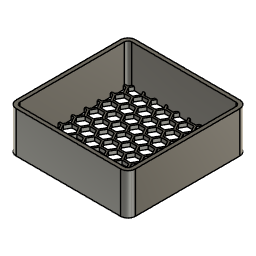
hex napkin holder v1.5 (Autodesk Fusion 360 design; units mm, degrees)
Autodesk Fusion 360 part; units mm, degrees
(part 1 of 14)
sketch "Sketch1" plane through (0, 0, 0) normal (0, 0, 1) x (1, 0, 0)
  line L0 (0, 0) -> (190.5, 0)
  line L1 (190.5, 0) -> (190.5, 190.5)
  line L2 (190.5, 190.5) -> (0, 190.5)
  line L3 (0, 190.5) -> (0, 0)
  line L4 (-6.35, -6.35) -> (196.85, -6.35)
  line L5 (196.85, -6.35) -> (196.85, 196.85)
  line L6 (196.85, 196.85) -> (-6.35, 196.85)
  line L7 (-6.35, 196.85) -> (-6.35, -6.35)
  point P0 (-273.976, 103.1875)
  dimension "d1" = 190.5
  dimension "d2" = 190.5
  dimension "d3" = 6.35
  constraint horizontal L0
  constraint vertical L1
  constraint horizontal L2
  constraint vertical L3
  constraint coincident L0.start L3.end
  measures "d1" distance of L0.start L0.end
  measures "d2" distance of L0.start L2.end
extrude "Extrude1" add sketch "Sketch1" along normal blind 6.35 contours L0 L1 L2 L3
extrude "Extrude2" add sketch "Sketch1" along normal blind 69.85
sketch "Sketch2" plane through (0, 0, 6.35) normal (0, 0, 1) x (-1, 0, 0)
  line L0 (0, -190.5) -> (0, 0)
  line L1 (0, 0) -> (-190.5, 0)
  line L2 (-190.5, 0) -> (-190.5, -190.5)
  line L3 (-190.5, -190.5) -> (0, -190.5)
  line L4 (-190.5, 0) -> (0, -190.5) construction
  line L5 (-190.5, -190.5) -> (0, 0) construction
  line L6 (-100.7493, -104.775) -> (-89.7507, -104.775)
  line L7 (-89.7507, -104.775) -> (-84.2515, -95.25)
  line L8 (-84.2515, -95.25) -> (-89.7507, -85.725)
  line L9 (-89.7507, -85.725) -> (-100.7493, -85.725)
  line L10 (-100.7493, -85.725) -> (-106.2485, -95.25)
  line L11 (-106.2485, -95.25) -> (-100.7493, -104.775)
  line L12 (-95.25, -95.25) -> (-151.2697, -192.279) construction
  line L13 (-95.25, -95.25) -> (-80.5853, -95.25) construction
  line L14 (-95.25, -95.25) -> (-103.4989, -100.0125) construction
  line L15 (-95.25, -95.25) -> (-87.0011, -100.0125) construction
  line L16 (-100.7493, 50.8) -> (-89.7507, 50.8)
  line L17 (-89.7507, 50.8) -> (-84.2515, 60.325)
  line L18 (-84.2515, 60.325) -> (-89.7507, 69.85)
  line L19 (-89.7507, 69.85) -> (-100.7493, 69.85)
  line L20 (-106.2485, 60.325) -> (-100.7493, 50.8)
  line L21 (-100.7493, 69.85) -> (-106.2485, 60.325)
  line L22 (-119.9967, 39.6875) -> (-108.9982, 39.6875)
  line L23 (-108.9982, 39.6875) -> (-103.4989, 49.2125)
  line L24 (-103.4989, 49.2125) -> (-108.9982, 58.7375)
  line L25 (-108.9982, 58.7375) -> (-119.9967, 58.7375)
  line L26 (-125.4959, 49.2125) -> (-119.9967, 39.6875)
  line L27 (-119.9967, 58.7375) -> (-125.4959, 49.2125)
  line L28 (-139.2441, 28.575) -> (-128.2456, 28.575)
  line L29 (-128.2456, 28.575) -> (-122.7463, 38.1)
  line L30 (-122.7463, 38.1) -> (-128.2456, 47.625)
  line L31 (-128.2456, 47.625) -> (-139.2441, 47.625)
  line L32 (-144.7434, 38.1) -> (-139.2441, 28.575)
  line L33 (-139.2441, 47.625) -> (-144.7434, 38.1)
  line L34 (-158.4915, 17.4625) -> (-147.493, 17.4625)
  line L35 (-147.493, 17.4625) -> (-141.9937, 26.9875)
  line L36 (-141.9937, 26.9875) -> (-147.493, 36.5125)
  line L37 (-147.493, 36.5125) -> (-158.4915, 36.5125)
  line L38 (-163.9908, 26.9875) -> (-158.4915, 17.4625)
  line L39 (-158.4915, 36.5125) -> (-163.9908, 26.9875)
  line L40 (-177.7389, 6.35) -> (-166.7404, 6.35)
  line L41 (-166.7404, 6.35) -> (-161.2411, 15.875)
  line L42 (-161.2411, 15.875) -> (-166.7404, 25.4)
  line L43 (-166.7404, 25.4) -> (-177.7389, 25.4)
  line L44 (-183.2382, 15.875) -> (-177.7389, 6.35)
  line L45 (-177.7389, 25.4) -> (-183.2382, 15.875)
  line L46 (-196.9863, -4.7625) -> (-185.9878, -4.7625)
  line L47 (-185.9878, -4.7625) -> (-180.4886, 4.7625)
  line L48 (-180.4886, 4.7625) -> (-185.9878, 14.2875)
  line L49 (-185.9878, 14.2875) -> (-196.9863, 14.2875)
  line L50 (-202.4856, 4.7625) -> (-196.9863, -4.7625)
  line L51 (-196.9863, 14.2875) -> (-202.4856, 4.7625)
  line L52 (-216.2337, -15.875) -> (-205.2352, -15.875)
  line L53 (-205.2352, -15.875) -> (-199.736, -6.35)
  line L54 (-199.736, -6.35) -> (-205.2352, 3.175)
  line L55 (-205.2352, 3.175) -> (-216.2337, 3.175)
  line L56 (-221.733, -6.35) -> (-216.2337, -15.875)
  line L57 (-216.2337, 3.175) -> (-221.733, -6.35)
  line L58 (-235.4812, -26.9875) -> (-224.4826, -26.9875)
  line L59 (-224.4826, -26.9875) -> (-218.9834, -17.4625)
  line L60 (-218.9834, -17.4625) -> (-224.4826, -7.9375)
  line L61 (-224.4826, -7.9375) -> (-235.4812, -7.9375)
  line L62 (-240.9804, -17.4625) -> (-235.4812, -26.9875)
  line L63 (-235.4812, -7.9375) -> (-240.9804, -17.4625)
  line L64 (-254.7286, -38.1) -> (-243.7301, -38.1)
  line L65 (-243.7301, -38.1) -> (-238.2308, -28.575)
  line L66 (-238.2308, -28.575) -> (-243.7301, -19.05)
  line L67 (-243.7301, -19.05) -> (-254.7286, -19.05)
  line L68 (-260.2278, -28.575) -> (-254.7286, -38.1)
  line L69 (-254.7286, -19.05) -> (-260.2278, -28.575)
  line L70 (-273.976, -49.2125) -> (-262.9775, -49.2125)
  line L71 (-262.9775, -49.2125) -> (-257.4782, -39.6875)
  line L72 (-257.4782, -39.6875) -> (-262.9775, -30.1625)
  line L73 (-262.9775, -30.1625) -> (-273.976, -30.1625)
  line L74 (-279.4753, -39.6875) -> (-273.976, -49.2125)
  line L75 (-273.976, -30.1625) -> (-279.4753, -39.6875)
  line L76 (-293.2234, -60.325) -> (-282.2249, -60.325)
  line L77 (-282.2249, -60.325) -> (-276.7256, -50.8)
  line L78 (-276.7256, -50.8) -> (-282.2249, -41.275)
  line L79 (-282.2249, -41.275) -> (-293.2234, -41.275)
  line L80 (-298.7227, -50.8) -> (-293.2234, -60.325)
  line L81 (-293.2234, -41.275) -> (-298.7227, -50.8)
  line L82 (-312.4708, -71.4375) -> (-301.4723, -71.4375)
  line L83 (-301.4723, -71.4375) -> (-295.973, -61.9125)
  line L84 (-295.973, -61.9125) -> (-301.4723, -52.3875)
  line L85 (-301.4723, -52.3875) -> (-312.4708, -52.3875)
  line L86 (-317.9701, -61.9125) -> (-312.4708, -71.4375)
  line L87 (-312.4708, -52.3875) -> (-317.9701, -61.9125)
  line L88 (-331.7182, -82.55) -> (-320.7197, -82.55)
  line L89 (-320.7197, -82.55) -> (-315.2205, -73.025)
  line L90 (-315.2205, -73.025) -> (-320.7197, -63.5)
  line L91 (-320.7197, -63.5) -> (-331.7182, -63.5)
  line L92 (-337.2175, -73.025) -> (-331.7182, -82.55)
  line L93 (-331.7182, -63.5) -> (-337.2175, -73.025)
  line L94 (-350.9657, -93.6625) -> (-339.9671, -93.6625)
  line L95 (-339.9671, -93.6625) -> (-334.4679, -84.1375)
  line L96 (-334.4679, -84.1375) -> (-339.9671, -74.6125)
  line L97 (-339.9671, -74.6125) -> (-350.9657, -74.6125)
  line L98 (-356.4649, -84.1375) -> (-350.9657, -93.6625)
  line L99 (-350.9657, -74.6125) -> (-356.4649, -84.1375)
  line L100 (-370.2131, -104.775) -> (-359.2145, -104.775)
  line L101 (-359.2145, -104.775) -> (-353.7153, -95.25)
  line L102 (-353.7153, -95.25) -> (-359.2145, -85.725)
  line L103 (-359.2145, -85.725) -> (-370.2131, -85.725)
  line L104 (-375.7123, -95.25) -> (-370.2131, -104.775)
  line L105 (-370.2131, -85.725) -> (-375.7123, -95.25)
  line L106 (-81.5018, 39.6875) -> (-70.5033, 39.6875)
  line L107 (-70.5033, 39.6875) -> (-65.0041, 49.2125)
  line L108 (-65.0041, 49.2125) -> (-70.5033, 58.7375)
  line L109 (-70.5033, 58.7375) -> (-81.5018, 58.7375)
  line L110 (-87.0011, 49.2125) -> (-81.5018, 39.6875)
  line L111 (-81.5018, 58.7375) -> (-87.0011, 49.2125)
  line L112 (-100.7493, 28.575) -> (-89.7507, 28.575)
  line L113 (-89.7507, 28.575) -> (-84.2515, 38.1)
  line L114 (-84.2515, 38.1) -> (-89.7507, 47.625)
  line L115 (-89.7507, 47.625) -> (-100.7493, 47.625)
  line L116 (-106.2485, 38.1) -> (-100.7493, 28.575)
  line L117 (-100.7493, 47.625) -> (-106.2485, 38.1)
  line L118 (-119.9967, 17.4625) -> (-108.9982, 17.4625)
  line L119 (-108.9982, 17.4625) -> (-103.4989, 26.9875)
  line L120 (-103.4989, 26.9875) -> (-108.9982, 36.5125)
  line L121 (-108.9982, 36.5125) -> (-119.9967, 36.5125)
  line L122 (-125.4959, 26.9875) -> (-119.9967, 17.4625)
  line L123 (-119.9967, 36.5125) -> (-125.4959, 26.9875)
  line L124 (-139.2441, 6.35) -> (-128.2456, 6.35)
  line L125 (-128.2456, 6.35) -> (-122.7463, 15.875)
  line L126 (-122.7463, 15.875) -> (-128.2456, 25.4)
  line L127 (-128.2456, 25.4) -> (-139.2441, 25.4)
  line L128 (-144.7434, 15.875) -> (-139.2441, 6.35)
  line L129 (-139.2441, 25.4) -> (-144.7434, 15.875)
  line L130 (-158.4915, -4.7625) -> (-147.493, -4.7625)
  line L131 (-147.493, -4.7625) -> (-141.9937, 4.7625)
  line L132 (-141.9937, 4.7625) -> (-147.493, 14.2875)
  line L133 (-147.493, 14.2875) -> (-158.4915, 14.2875)
  line L134 (-163.9908, 4.7625) -> (-158.4915, -4.7625)
  line L135 (-158.4915, 14.2875) -> (-163.9908, 4.7625)
  line L136 (-177.7389, -15.875) -> (-166.7404, -15.875)
  line L137 (-166.7404, -15.875) -> (-161.2411, -6.35)
  line L138 (-161.2411, -6.35) -> (-166.7404, 3.175)
  line L139 (-166.7404, 3.175) -> (-177.7389, 3.175)
  line L140 (-183.2382, -6.35) -> (-177.7389, -15.875)
  line L141 (-177.7389, 3.175) -> (-183.2382, -6.35)
  line L142 (-196.9863, -26.9875) -> (-185.9878, -26.9875)
  line L143 (-185.9878, -26.9875) -> (-180.4886, -17.4625)
  line L144 (-180.4886, -17.4625) -> (-185.9878, -7.9375)
  line L145 (-185.9878, -7.9375) -> (-196.9863, -7.9375)
  line L146 (-202.4856, -17.4625) -> (-196.9863, -26.9875)
  line L147 (-196.9863, -7.9375) -> (-202.4856, -17.4625)
  line L148 (-216.2337, -38.1) -> (-205.2352, -38.1)
  line L149 (-205.2352, -38.1) -> (-199.736, -28.575)
  line L150 (-199.736, -28.575) -> (-205.2352, -19.05)
  line L151 (-205.2352, -19.05) -> (-216.2337, -19.05)
  line L152 (-221.733, -28.575) -> (-216.2337, -38.1)
  line L153 (-216.2337, -19.05) -> (-221.733, -28.575)
  line L154 (-235.4812, -49.2125) -> (-224.4826, -49.2125)
  line L155 (-224.4826, -49.2125) -> (-218.9834, -39.6875)
  line L156 (-218.9834, -39.6875) -> (-224.4826, -30.1625)
  line L157 (-224.4826, -30.1625) -> (-235.4812, -30.1625)
  line L158 (-240.9804, -39.6875) -> (-235.4812, -49.2125)
  line L159 (-235.4812, -30.1625) -> (-240.9804, -39.6875)
  line L160 (-254.7286, -60.325) -> (-243.7301, -60.325)
  line L161 (-243.7301, -60.325) -> (-238.2308, -50.8)
  line L162 (-238.2308, -50.8) -> (-243.7301, -41.275)
  line L163 (-243.7301, -41.275) -> (-254.7286, -41.275)
  line L164 (-260.2278, -50.8) -> (-254.7286, -60.325)
  line L165 (-254.7286, -41.275) -> (-260.2278, -50.8)
  line L166 (-273.976, -71.4375) -> (-262.9775, -71.4375)
  line L167 (-262.9775, -71.4375) -> (-257.4782, -61.9125)
  line L168 (-257.4782, -61.9125) -> (-262.9775, -52.3875)
  line L169 (-262.9775, -52.3875) -> (-273.976, -52.3875)
  line L170 (-279.4753, -61.9125) -> (-273.976, -71.4375)
  line L171 (-273.976, -52.3875) -> (-279.4753, -61.9125)
  line L172 (-293.2234, -82.55) -> (-282.2249, -82.55)
  line L173 (-282.2249, -82.55) -> (-276.7256, -73.025)
  line L174 (-276.7256, -73.025) -> (-282.2249, -63.5)
  line L175 (-282.2249, -63.5) -> (-293.2234, -63.5)
  line L176 (-298.7227, -73.025) -> (-293.2234, -82.55)
  line L177 (-293.2234, -63.5) -> (-298.7227, -73.025)
  line L178 (-312.4708, -93.6625) -> (-301.4723, -93.6625)
  line L179 (-301.4723, -93.6625) -> (-295.973, -84.1375)
  line L180 (-295.973, -84.1375) -> (-301.4723, -74.6125)
  line L181 (-301.4723, -74.6125) -> (-312.4708, -74.6125)
  line L182 (-317.9701, -84.1375) -> (-312.4708, -93.6625)
  line L183 (-312.4708, -74.6125) -> (-317.9701, -84.1375)
  line L184 (-331.7182, -104.775) -> (-320.7197, -104.775)
  line L185 (-320.7197, -104.775) -> (-315.2205, -95.25)
  line L186 (-315.2205, -95.25) -> (-320.7197, -85.725)
  line L187 (-320.7197, -85.725) -> (-331.7182, -85.725)
  line L188 (-337.2175, -95.25) -> (-331.7182, -104.775)
  line L189 (-331.7182, -85.725) -> (-337.2175, -95.25)
  line L190 (-350.9657, -115.8875) -> (-339.9671, -115.8875)
  line L191 (-339.9671, -115.8875) -> (-334.4679, -106.3625)
  line L192 (-334.4679, -106.3625) -> (-339.9671, -96.8375)
  line L193 (-339.9671, -96.8375) -> (-350.9657, -96.8375)
  line L194 (-356.4649, -106.3625) -> (-350.9657, -115.8875)
  line L195 (-350.9657, -96.8375) -> (-356.4649, -106.3625)
  line L196 (-62.2544, 28.575) -> (-51.2559, 28.575)
  line L197 (-51.2559, 28.575) -> (-45.7566, 38.1)
  line L198 (-45.7566, 38.1) -> (-51.2559, 47.625)
  line L199 (-51.2559, 47.625) -> (-62.2544, 47.625)
  line L200 (-67.7537, 38.1) -> (-62.2544, 28.575)
  line L201 (-62.2544, 47.625) -> (-67.7537, 38.1)
  line L202 (-81.5018, 17.4625) -> (-70.5033, 17.4625)
  line L203 (-70.5033, 17.4625) -> (-65.0041, 26.9875)
  line L204 (-65.0041, 26.9875) -> (-70.5033, 36.5125)
  line L205 (-70.5033, 36.5125) -> (-81.5018, 36.5125)
  line L206 (-87.0011, 26.9875) -> (-81.5018, 17.4625)
  line L207 (-81.5018, 36.5125) -> (-87.0011, 26.9875)
  line L208 (-100.7493, 6.35) -> (-89.7507, 6.35)
  line L209 (-89.7507, 6.35) -> (-84.2515, 15.875)
  line L210 (-84.2515, 15.875) -> (-89.7507, 25.4)
  line L211 (-89.7507, 25.4) -> (-100.7493, 25.4)
  line L212 (-106.2485, 15.875) -> (-100.7493, 6.35)
  line L213 (-100.7493, 25.4) -> (-106.2485, 15.875)
  line L214 (-119.9967, -4.7625) -> (-108.9982, -4.7625)
  line L215 (-108.9982, -4.7625) -> (-103.4989, 4.7625)
  line L216 (-103.4989, 4.7625) -> (-108.9982, 14.2875)
  line L217 (-108.9982, 14.2875) -> (-119.9967, 14.2875)
  line L218 (-125.4959, 4.7625) -> (-119.9967, -4.7625)
  line L219 (-119.9967, 14.2875) -> (-125.4959, 4.7625)
  line L220 (-139.2441, -15.875) -> (-128.2456, -15.875)
  line L221 (-128.2456, -15.875) -> (-122.7463, -6.35)
  line L222 (-122.7463, -6.35) -> (-128.2456, 3.175)
  line L223 (-128.2456, 3.175) -> (-139.2441, 3.175)
  line L224 (-144.7434, -6.35) -> (-139.2441, -15.875)
  line L225 (-139.2441, 3.175) -> (-144.7434, -6.35)
  line L226 (-158.4915, -26.9875) -> (-147.493, -26.9875)
  line L227 (-147.493, -26.9875) -> (-141.9937, -17.4625)
  line L228 (-141.9937, -17.4625) -> (-147.493, -7.9375)
  line L229 (-147.493, -7.9375) -> (-158.4915, -7.9375)
  line L230 (-163.9908, -17.4625) -> (-158.4915, -26.9875)
  line L231 (-158.4915, -7.9375) -> (-163.9908, -17.4625)
  line L232 (-177.7389, -38.1) -> (-166.7404, -38.1)
  line L233 (-166.7404, -38.1) -> (-161.2411, -28.575)
  line L234 (-161.2411, -28.575) -> (-166.7404, -19.05)
  line L235 (-166.7404, -19.05) -> (-177.7389, -19.05)
  line L236 (-183.2382, -28.575) -> (-177.7389, -38.1)
  line L237 (-177.7389, -19.05) -> (-183.2382, -28.575)
  line L238 (-196.9863, -49.2125) -> (-185.9878, -49.2125)
  line L239 (-185.9878, -49.2125) -> (-180.4886, -39.6875)
  line L240 (-180.4886, -39.6875) -> (-185.9878, -30.1625)
  line L241 (-185.9878, -30.1625) -> (-196.9863, -30.1625)
  line L242 (-202.4856, -39.6875) -> (-196.9863, -49.2125)
  line L243 (-196.9863, -30.1625) -> (-202.4856, -39.6875)
  line L244 (-216.2337, -60.325) -> (-205.2352, -60.325)
  line L245 (-205.2352, -60.325) -> (-199.736, -50.8)
  line L246 (-199.736, -50.8) -> (-205.2352, -41.275)
  line L247 (-205.2352, -41.275) -> (-216.2337, -41.275)
  line L248 (-221.733, -50.8) -> (-216.2337, -60.325)
  line L249 (-216.2337, -41.275) -> (-221.733, -50.8)
  line L250 (-235.4812, -71.4375) -> (-224.4826, -71.4375)
  line L251 (-224.4826, -71.4375) -> (-218.9834, -61.9125)
  line L252 (-218.9834, -61.9125) -> (-224.4826, -52.3875)
  line L253 (-224.4826, -52.3875) -> (-235.4812, -52.3875)
  line L254 (-240.9804, -61.9125) -> (-235.4812, -71.4375)
  line L255 (-235.4812, -52.3875) -> (-240.9804, -61.9125)
  line L256 (-254.7286, -82.55) -> (-243.7301, -82.55)
  line L257 (-243.7301, -82.55) -> (-238.2308, -73.025)
  line L258 (-238.2308, -73.025) -> (-243.7301, -63.5)
  line L259 (-243.7301, -63.5) -> (-254.7286, -63.5)
  line L260 (-260.2278, -73.025) -> (-254.7286, -82.55)
  line L261 (-254.7286, -63.5) -> (-260.2278, -73.025)
  line L262 (-273.976, -93.6625) -> (-262.9775, -93.6625)
  line L263 (-262.9775, -93.6625) -> (-257.4782, -84.1375)
  line L264 (-257.4782, -84.1375) -> (-262.9775, -74.6125)
  line L265 (-262.9775, -74.6125) -> (-273.976, -74.6125)
  line L266 (-279.4753, -84.1375) -> (-273.976, -93.6625)
  line L267 (-273.976, -74.6125) -> (-279.4753, -84.1375)
  line L268 (-293.2234, -104.775) -> (-282.2249, -104.775)
  line L269 (-282.2249, -104.775) -> (-276.7256, -95.25)
  line L270 (-276.7256, -95.25) -> (-282.2249, -85.725)
  line L271 (-282.2249, -85.725) -> (-293.2234, -85.725)
  line L272 (-298.7227, -95.25) -> (-293.2234, -104.775)
  line L273 (-293.2234, -85.725) -> (-298.7227, -95.25)
  line L274 (-312.4708, -115.8875) -> (-301.4723, -115.8875)
  line L275 (-301.4723, -115.8875) -> (-295.973, -106.3625)
  line L276 (-295.973, -106.3625) -> (-301.4723, -96.8375)
  line L277 (-301.4723, -96.8375) -> (-312.4708, -96.8375)
  line L278 (-317.9701, -106.3625) -> (-312.4708, -115.8875)
  line L279 (-312.4708, -96.8375) -> (-317.9701, -106.3625)
  line L280 (-331.7182, -127) -> (-320.7197, -127)
  line L281 (-320.7197, -127) -> (-315.2205, -117.475)
  line L282 (-315.2205, -117.475) -> (-320.7197, -107.95)
  line L283 (-320.7197, -107.95) -> (-331.7182, -107.95)
  line L284 (-337.2175, -117.475) -> (-331.7182, -127)
  line L285 (-331.7182, -107.95) -> (-337.2175, -117.475)
  line L286 (-43.007, 17.4625) -> (-32.0085, 17.4625)
  line L287 (-32.0085, 17.4625) -> (-26.5092, 26.9875)
  line L288 (-26.5092, 26.9875) -> (-32.0085, 36.5125)
  line L289 (-32.0085, 36.5125) -> (-43.007, 36.5125)
  line L290 (-48.5063, 26.9875) -> (-43.007, 17.4625)
  line L291 (-43.007, 36.5125) -> (-48.5063, 26.9875)
  line L292 (-62.2544, 6.35) -> (-51.2559, 6.35)
  line L293 (-51.2559, 6.35) -> (-45.7566, 15.875)
  line L294 (-45.7566, 15.875) -> (-51.2559, 25.4)
  line L295 (-51.2559, 25.4) -> (-62.2544, 25.4)
  line L296 (-67.7537, 15.875) -> (-62.2544, 6.35)
  line L297 (-62.2544, 25.4) -> (-67.7537, 15.875)
  line L298 (-81.5018, -4.7625) -> (-70.5033, -4.7625)
  line L299 (-70.5033, -4.7625) -> (-65.0041, 4.7625)
  line L300 (-65.0041, 4.7625) -> (-70.5033, 14.2875)
  line L301 (-70.5033, 14.2875) -> (-81.5018, 14.2875)
  line L302 (-87.0011, 4.7625) -> (-81.5018, -4.7625)
  line L303 (-81.5018, 14.2875) -> (-87.0011, 4.7625)
  line L304 (-100.7493, -15.875) -> (-89.7507, -15.875)
  line L305 (-89.7507, -15.875) -> (-84.2515, -6.35)
  line L306 (-84.2515, -6.35) -> (-89.7507, 3.175)
  line L307 (-89.7507, 3.175) -> (-100.7493, 3.175)
  line L308 (-106.2485, -6.35) -> (-100.7493, -15.875)
  line L309 (-100.7493, 3.175) -> (-106.2485, -6.35)
  line L310 (-119.9967, -26.9875) -> (-108.9982, -26.9875)
  line L311 (-108.9982, -26.9875) -> (-103.4989, -17.4625)
  line L312 (-103.4989, -17.4625) -> (-108.9982, -7.9375)
  line L313 (-108.9982, -7.9375) -> (-119.9967, -7.9375)
  line L314 (-125.4959, -17.4625) -> (-119.9967, -26.9875)
  line L315 (-119.9967, -7.9375) -> (-125.4959, -17.4625)
  line L316 (-139.2441, -38.1) -> (-128.2456, -38.1)
  line L317 (-128.2456, -38.1) -> (-122.7463, -28.575)
  line L318 (-122.7463, -28.575) -> (-128.2456, -19.05)
  line L319 (-128.2456, -19.05) -> (-139.2441, -19.05)
  line L320 (-144.7434, -28.575) -> (-139.2441, -38.1)
  line L321 (-139.2441, -19.05) -> (-144.7434, -28.575)
  line L322 (-158.4915, -49.2125) -> (-147.493, -49.2125)
  line L323 (-147.493, -49.2125) -> (-141.9937, -39.6875)
  line L324 (-141.9937, -39.6875) -> (-147.493, -30.1625)
  line L325 (-147.493, -30.1625) -> (-158.4915, -30.1625)
  line L326 (-163.9908, -39.6875) -> (-158.4915, -49.2125)
  line L327 (-158.4915, -30.1625) -> (-163.9908, -39.6875)
  line L328 (-177.7389, -60.325) -> (-166.7404, -60.325)
  line L329 (-166.7404, -60.325) -> (-161.2411, -50.8)
  line L330 (-161.2411, -50.8) -> (-166.7404, -41.275)
  line L331 (-166.7404, -41.275) -> (-177.7389, -41.275)
  line L332 (-183.2382, -50.8) -> (-177.7389, -60.325)
  line L333 (-177.7389, -41.275) -> (-183.2382, -50.8)
  line L334 (-196.9863, -71.4375) -> (-185.9878, -71.4375)
  line L335 (-185.9878, -71.4375) -> (-180.4886, -61.9125)
  line L336 (-180.4886, -61.9125) -> (-185.9878, -52.3875)
  line L337 (-185.9878, -52.3875) -> (-196.9863, -52.3875)
  line L338 (-202.4856, -61.9125) -> (-196.9863, -71.4375)
  line L339 (-196.9863, -52.3875) -> (-202.4856, -61.9125)
  line L340 (-216.2337, -82.55) -> (-205.2352, -82.55)
  line L341 (-205.2352, -82.55) -> (-199.736, -73.025)
  line L342 (-199.736, -73.025) -> (-205.2352, -63.5)
  line L343 (-205.2352, -63.5) -> (-216.2337, -63.5)
  line L344 (-221.733, -73.025) -> (-216.2337, -82.55)
  line L345 (-216.2337, -63.5) -> (-221.733, -73.025)
  line L346 (-235.4812, -93.6625) -> (-224.4826, -93.6625)
  line L347 (-224.4826, -93.6625) -> (-218.9834, -84.1375)
  line L348 (-218.9834, -84.1375) -> (-224.4826, -74.6125)
  line L349 (-224.4826, -74.6125) -> (-235.4812, -74.6125)
  line L350 (-240.9804, -84.1375) -> (-235.4812, -93.6625)
  line L351 (-235.4812, -74.6125) -> (-240.9804, -84.1375)
  line L352 (-254.7286, -104.775) -> (-243.7301, -104.775)
  line L353 (-243.7301, -104.775) -> (-238.2308, -95.25)
  line L354 (-238.2308, -95.25) -> (-243.7301, -85.725)
  line L355 (-243.7301, -85.725) -> (-254.7286, -85.725)
  line L356 (-260.2278, -95.25) -> (-254.7286, -104.775)
  line L357 (-254.7286, -85.725) -> (-260.2278, -95.25)
  line L358 (-273.976, -115.8875) -> (-262.9775, -115.8875)
  line L359 (-262.9775, -115.8875) -> (-257.4782, -106.3625)
  line L360 (-257.4782, -106.3625) -> (-262.9775, -96.8375)
  line L361 (-262.9775, -96.8375) -> (-273.976, -96.8375)
  line L362 (-279.4753, -106.3625) -> (-273.976, -115.8875)
  line L363 (-273.976, -96.8375) -> (-279.4753, -106.3625)
  line L364 (-293.2234, -127) -> (-282.2249, -127)
  line L365 (-282.2249, -127) -> (-276.7256, -117.475)
  line L366 (-276.7256, -117.475) -> (-282.2249, -107.95)
  line L367 (-282.2249, -107.95) -> (-293.2234, -107.95)
  line L368 (-298.7227, -117.475) -> (-293.2234, -127)
  line L369 (-293.2234, -107.95) -> (-298.7227, -117.475)
  line L370 (-312.4708, -138.1125) -> (-301.4723, -138.1125)
  line L371 (-301.4723, -138.1125) -> (-295.973, -128.5875)
  line L372 (-295.973, -128.5875) -> (-301.4723, -119.0625)
  line L373 (-301.4723, -119.0625) -> (-312.4708, -119.0625)
  line L374 (-317.9701, -128.5875) -> (-312.4708, -138.1125)
  line L375 (-312.4708, -119.0625) -> (-317.9701, -128.5875)
  line L376 (-23.7596, 6.35) -> (-12.7611, 6.35)
  line L377 (-12.7611, 6.35) -> (-7.2618, 15.875)
  line L378 (-7.2618, 15.875) -> (-12.7611, 25.4)
  line L379 (-12.7611, 25.4) -> (-23.7596, 25.4)
  line L380 (-29.2589, 15.875) -> (-23.7596, 6.35)
  line L381 (-23.7596, 25.4) -> (-29.2589, 15.875)
  line L382 (-43.007, -4.7625) -> (-32.0085, -4.7625)
  line L383 (-32.0085, -4.7625) -> (-26.5092, 4.7625)
  line L384 (-26.5092, 4.7625) -> (-32.0085, 14.2875)
  line L385 (-32.0085, 14.2875) -> (-43.007, 14.2875)
  line L386 (-48.5063, 4.7625) -> (-43.007, -4.7625)
  line L387 (-43.007, 14.2875) -> (-48.5063, 4.7625)
  line L388 (-62.2544, -15.875) -> (-51.2559, -15.875)
  line L389 (-51.2559, -15.875) -> (-45.7566, -6.35)
  line L390 (-45.7566, -6.35) -> (-51.2559, 3.175)
  line L391 (-51.2559, 3.175) -> (-62.2544, 3.175)
  line L392 (-67.7537, -6.35) -> (-62.2544, -15.875)
  line L393 (-62.2544, 3.175) -> (-67.7537, -6.35)
  line L394 (-81.5018, -26.9875) -> (-70.5033, -26.9875)
  line L395 (-70.5033, -26.9875) -> (-65.0041, -17.4625)
  line L396 (-65.0041, -17.4625) -> (-70.5033, -7.9375)
  line L397 (-70.5033, -7.9375) -> (-81.5018, -7.9375)
  line L398 (-87.0011, -17.4625) -> (-81.5018, -26.9875)
  line L399 (-81.5018, -7.9375) -> (-87.0011, -17.4625)
  line L400 (-100.7493, -38.1) -> (-89.7507, -38.1)
  line L401 (-89.7507, -38.1) -> (-84.2515, -28.575)
  line L402 (-84.2515, -28.575) -> (-89.7507, -19.05)
  line L403 (-89.7507, -19.05) -> (-100.7493, -19.05)
  line L404 (-106.2485, -28.575) -> (-100.7493, -38.1)
  line L405 (-100.7493, -19.05) -> (-106.2485, -28.575)
  line L406 (-119.9967, -49.2125) -> (-108.9982, -49.2125)
  line L407 (-108.9982, -49.2125) -> (-103.4989, -39.6875)
  line L408 (-103.4989, -39.6875) -> (-108.9982, -30.1625)
  line L409 (-108.9982, -30.1625) -> (-119.9967, -30.1625)
  line L410 (-125.4959, -39.6875) -> (-119.9967, -49.2125)
  line L411 (-119.9967, -30.1625) -> (-125.4959, -39.6875)
  line L412 (-139.2441, -60.325) -> (-128.2456, -60.325)
  line L413 (-128.2456, -60.325) -> (-122.7463, -50.8)
  line L414 (-122.7463, -50.8) -> (-128.2456, -41.275)
  line L415 (-128.2456, -41.275) -> (-139.2441, -41.275)
  line L416 (-144.7434, -50.8) -> (-139.2441, -60.325)
  line L417 (-139.2441, -41.275) -> (-144.7434, -50.8)
  line L418 (-158.4915, -71.4375) -> (-147.493, -71.4375)
  line L419 (-147.493, -71.4375) -> (-141.9937, -61.9125)
  line L420 (-141.9937, -61.9125) -> (-147.493, -52.3875)
  line L421 (-147.493, -52.3875) -> (-158.4915, -52.3875)
  line L422 (-163.9908, -61.9125) -> (-158.4915, -71.4375)
  line L423 (-158.4915, -52.3875) -> (-163.9908, -61.9125)
  line L424 (-177.7389, -82.55) -> (-166.7404, -82.55)
  line L425 (-166.7404, -82.55) -> (-161.2411, -73.025)
  line L426 (-161.2411, -73.025) -> (-166.7404, -63.5)
  line L427 (-166.7404, -63.5) -> (-177.7389, -63.5)
  line L428 (-183.2382, -73.025) -> (-177.7389, -82.55)
  line L429 (-177.7389, -63.5) -> (-183.2382, -73.025)
  line L430 (-196.9863, -93.6625) -> (-185.9878, -93.6625)
  line L431 (-185.9878, -93.6625) -> (-180.4886, -84.1375)
  line L432 (-180.4886, -84.1375) -> (-185.9878, -74.6125)
  line L433 (-185.9878, -74.6125) -> (-196.9863, -74.6125)
  line L434 (-202.4856, -84.1375) -> (-196.9863, -93.6625)
  line L435 (-196.9863, -74.6125) -> (-202.4856, -84.1375)
  line L436 (-216.2337, -104.775) -> (-205.2352, -104.775)
  line L437 (-205.2352, -104.775) -> (-199.736, -95.25)
  line L438 (-199.736, -95.25) -> (-205.2352, -85.725)
  line L439 (-205.2352, -85.725) -> (-216.2337, -85.725)
  line L440 (-221.733, -95.25) -> (-216.2337, -104.775)
  line L441 (-216.2337, -85.725) -> (-221.733, -95.25)
  line L442 (-235.4812, -115.8875) -> (-224.4826, -115.8875)
  line L443 (-224.4826, -115.8875) -> (-218.9834, -106.3625)
  line L444 (-218.9834, -106.3625) -> (-224.4826, -96.8375)
  line L445 (-224.4826, -96.8375) -> (-235.4812, -96.8375)
  line L446 (-240.9804, -106.3625) -> (-235.4812, -115.8875)
  line L447 (-235.4812, -96.8375) -> (-240.9804, -106.3625)
  line L448 (-254.7286, -127) -> (-243.7301, -127)
  line L449 (-243.7301, -127) -> (-238.2308, -117.475)
  line L450 (-238.2308, -117.475) -> (-243.7301, -107.95)
  line L451 (-243.7301, -107.95) -> (-254.7286, -107.95)
  line L452 (-260.2278, -117.475) -> (-254.7286, -127)
  line L453 (-254.7286, -107.95) -> (-260.2278, -117.475)
  line L454 (-273.976, -138.1125) -> (-262.9775, -138.1125)
  line L455 (-262.9775, -138.1125) -> (-257.4782, -128.5875)
  line L456 (-257.4782, -128.5875) -> (-262.9775, -119.0625)
  line L457 (-262.9775, -119.0625) -> (-273.976, -119.0625)
  line L458 (-279.4753, -128.5875) -> (-273.976, -138.1125)
  line L459 (-273.976, -119.0625) -> (-279.4753, -128.5875)
  line L460 (-293.2234, -149.225) -> (-282.2249, -149.225)
  line L461 (-282.2249, -149.225) -> (-276.7256, -139.7)
  line L462 (-276.7256, -139.7) -> (-282.2249, -130.175)
  line L463 (-282.2249, -130.175) -> (-293.2234, -130.175)
  line L464 (-298.7227, -139.7) -> (-293.2234, -149.225)
  line L465 (-293.2234, -130.175) -> (-298.7227, -139.7)
  line L466 (-4.5122, -4.7625) -> (6.4863, -4.7625)
  line L467 (6.4863, -4.7625) -> (11.9856, 4.7625)
  line L468 (11.9856, 4.7625) -> (6.4863, 14.2875)
  line L469 (6.4863, 14.2875) -> (-4.5122, 14.2875)
  line L470 (-10.0114, 4.7625) -> (-4.5122, -4.7625)
  line L471 (-4.5122, 14.2875) -> (-10.0114, 4.7625)
  line L472 (-23.7596, -15.875) -> (-12.7611, -15.875)
  line L473 (-12.7611, -15.875) -> (-7.2618, -6.35)
  line L474 (-7.2618, -6.35) -> (-12.7611, 3.175)
  line L475 (-12.7611, 3.175) -> (-23.7596, 3.175)
  line L476 (-29.2589, -6.35) -> (-23.7596, -15.875)
  line L477 (-23.7596, 3.175) -> (-29.2589, -6.35)
  line L478 (-43.007, -26.9875) -> (-32.0085, -26.9875)
  line L479 (-32.0085, -26.9875) -> (-26.5092, -17.4625)
  line L480 (-26.5092, -17.4625) -> (-32.0085, -7.9375)
  line L481 (-32.0085, -7.9375) -> (-43.007, -7.9375)
  line L482 (-48.5063, -17.4625) -> (-43.007, -26.9875)
  line L483 (-43.007, -7.9375) -> (-48.5063, -17.4625)
  line L484 (-62.2544, -38.1) -> (-51.2559, -38.1)
  line L485 (-51.2559, -38.1) -> (-45.7566, -28.575)
  line L486 (-45.7566, -28.575) -> (-51.2559, -19.05)
  line L487 (-51.2559, -19.05) -> (-62.2544, -19.05)
  line L488 (-67.7537, -28.575) -> (-62.2544, -38.1)
  line L489 (-62.2544, -19.05) -> (-67.7537, -28.575)
  line L490 (-81.5018, -49.2125) -> (-70.5033, -49.2125)
  line L491 (-70.5033, -49.2125) -> (-65.0041, -39.6875)
  line L492 (-65.0041, -39.6875) -> (-70.5033, -30.1625)
  line L493 (-70.5033, -30.1625) -> (-81.5018, -30.1625)
  line L494 (-87.0011, -39.6875) -> (-81.5018, -49.2125)
  line L495 (-81.5018, -30.1625) -> (-87.0011, -39.6875)
  line L496 (-100.7493, -60.325) -> (-89.7507, -60.325)
  line L497 (-89.7507, -60.325) -> (-84.2515, -50.8)
  line L498 (-84.2515, -50.8) -> (-89.7507, -41.275)
  line L499 (-89.7507, -41.275) -> (-100.7493, -41.275)
  line L500 (-106.2485, -50.8) -> (-100.7493, -60.325)
  line L501 (-100.7493, -41.275) -> (-106.2485, -50.8)
  line L502 (-119.9967, -71.4375) -> (-108.9982, -71.4375)
  line L503 (-108.9982, -71.4375) -> (-103.4989, -61.9125)
  line L504 (-103.4989, -61.9125) -> (-108.9982, -52.3875)
  line L505 (-108.9982, -52.3875) -> (-119.9967, -52.3875)
  line L506 (-125.4959, -61.9125) -> (-119.9967, -71.4375)
  line L507 (-119.9967, -52.3875) -> (-125.4959, -61.9125)
  line L508 (-139.2441, -82.55) -> (-128.2456, -82.55)
  line L509 (-128.2456, -82.55) -> (-122.7463, -73.025)
  line L510 (-122.7463, -73.025) -> (-128.2456, -63.5)
  line L511 (-128.2456, -63.5) -> (-139.2441, -63.5)
  line L512 (-144.7434, -73.025) -> (-139.2441, -82.55)
  line L513 (-139.2441, -63.5) -> (-144.7434, -73.025)
  line L514 (-158.4915, -93.6625) -> (-147.493, -93.6625)
  line L515 (-147.493, -93.6625) -> (-141.9937, -84.1375)
  line L516 (-141.9937, -84.1375) -> (-147.493, -74.6125)
  line L517 (-147.493, -74.6125) -> (-158.4915, -74.6125)
  line L518 (-163.9908, -84.1375) -> (-158.4915, -93.6625)
  line L519 (-158.4915, -74.6125) -> (-163.9908, -84.1375)
  line L520 (-177.7389, -104.775) -> (-166.7404, -104.775)
  line L521 (-166.7404, -104.775) -> (-161.2411, -95.25)
  line L522 (-161.2411, -95.25) -> (-166.7404, -85.725)
  line L523 (-166.7404, -85.725) -> (-177.7389, -85.725)
  line L524 (-183.2382, -95.25) -> (-177.7389, -104.775)
  line L525 (-177.7389, -85.725) -> (-183.2382, -95.25)
  line L526 (-196.9863, -115.8875) -> (-185.9878, -115.8875)
  line L527 (-185.9878, -115.8875) -> (-180.4886, -106.3625)
  line L528 (-180.4886, -106.3625) -> (-185.9878, -96.8375)
  line L529 (-185.9878, -96.8375) -> (-196.9863, -96.8375)
  line L530 (-202.4856, -106.3625) -> (-196.9863, -115.8875)
  line L531 (-196.9863, -96.8375) -> (-202.4856, -106.3625)
  line L532 (-216.2337, -127) -> (-205.2352, -127)
  line L533 (-205.2352, -127) -> (-199.736, -117.475)
  line L534 (-199.736, -117.475) -> (-205.2352, -107.95)
  line L535 (-205.2352, -107.95) -> (-216.2337, -107.95)
  line L536 (-221.733, -117.475) -> (-216.2337, -127)
  line L537 (-216.2337, -107.95) -> (-221.733, -117.475)
  line L538 (-235.4812, -138.1125) -> (-224.4826, -138.1125)
  line L539 (-224.4826, -138.1125) -> (-218.9834, -128.5875)
  line L540 (-218.9834, -128.5875) -> (-224.4826, -119.0625)
  line L541 (-224.4826, -119.0625) -> (-235.4812, -119.0625)
  line L542 (-240.9804, -128.5875) -> (-235.4812, -138.1125)
  line L543 (-235.4812, -119.0625) -> (-240.9804, -128.5875)
  line L544 (-254.7286, -149.225) -> (-243.7301, -149.225)
  line L545 (-243.7301, -149.225) -> (-238.2308, -139.7)
  line L546 (-238.2308, -139.7) -> (-243.7301, -130.175)
  line L547 (-243.7301, -130.175) -> (-254.7286, -130.175)
  line L548 (-260.2278, -139.7) -> (-254.7286, -149.225)
  line L549 (-254.7286, -130.175) -> (-260.2278, -139.7)
  line L550 (-273.976, -160.3375) -> (-262.9775, -160.3375)
  line L551 (-262.9775, -160.3375) -> (-257.4782, -150.8125)
  line L552 (-257.4782, -150.8125) -> (-262.9775, -141.2875)
  line L553 (-262.9775, -141.2875) -> (-273.976, -141.2875)
  line L554 (-279.4753, -150.8125) -> (-273.976, -160.3375)
  line L555 (-273.976, -141.2875) -> (-279.4753, -150.8125)
  line L556 (14.7352, -15.875) -> (25.7337, -15.875)
  line L557 (25.7337, -15.875) -> (31.233, -6.35)
  line L558 (31.233, -6.35) -> (25.7337, 3.175)
  line L559 (25.7337, 3.175) -> (14.7352, 3.175)
  line L560 (9.236, -6.35) -> (14.7352, -15.875)
  line L561 (14.7352, 3.175) -> (9.236, -6.35)
  line L562 (-4.5122, -26.9875) -> (6.4863, -26.9875)
  line L563 (6.4863, -26.9875) -> (11.9856, -17.4625)
  line L564 (11.9856, -17.4625) -> (6.4863, -7.9375)
  line L565 (6.4863, -7.9375) -> (-4.5122, -7.9375)
  line L566 (-10.0114, -17.4625) -> (-4.5122, -26.9875)
  line L567 (-4.5122, -7.9375) -> (-10.0114, -17.4625)
  line L568 (-23.7596, -38.1) -> (-12.7611, -38.1)
  line L569 (-12.7611, -38.1) -> (-7.2618, -28.575)
  line L570 (-7.2618, -28.575) -> (-12.7611, -19.05)
  line L571 (-12.7611, -19.05) -> (-23.7596, -19.05)
  line L572 (-29.2589, -28.575) -> (-23.7596, -38.1)
  line L573 (-23.7596, -19.05) -> (-29.2589, -28.575)
  line L574 (-43.007, -49.2125) -> (-32.0085, -49.2125)
  line L575 (-32.0085, -49.2125) -> (-26.5092, -39.6875)
  line L576 (-26.5092, -39.6875) -> (-32.0085, -30.1625)
  line L577 (-32.0085, -30.1625) -> (-43.007, -30.1625)
  line L578 (-48.5063, -39.6875) -> (-43.007, -49.2125)
  line L579 (-43.007, -30.1625) -> (-48.5063, -39.6875)
  line L580 (-62.2544, -60.325) -> (-51.2559, -60.325)
  line L581 (-51.2559, -60.325) -> (-45.7566, -50.8)
  line L582 (-45.7566, -50.8) -> (-51.2559, -41.275)
  line L583 (-51.2559, -41.275) -> (-62.2544, -41.275)
  line L584 (-67.7537, -50.8) -> (-62.2544, -60.325)
  line L585 (-62.2544, -41.275) -> (-67.7537, -50.8)
  line L586 (-81.5018, -71.4375) -> (-70.5033, -71.4375)
  line L587 (-70.5033, -71.4375) -> (-65.0041, -61.9125)
  line L588 (-65.0041, -61.9125) -> (-70.5033, -52.3875)
  line L589 (-70.5033, -52.3875) -> (-81.5018, -52.3875)
  line L590 (-87.0011, -61.9125) -> (-81.5018, -71.4375)
  line L591 (-81.5018, -52.3875) -> (-87.0011, -61.9125)
  line L592 (-100.7493, -82.55) -> (-89.7507, -82.55)
  line L593 (-89.7507, -82.55) -> (-84.2515, -73.025)
  line L594 (-84.2515, -73.025) -> (-89.7507, -63.5)
  line L595 (-89.7507, -63.5) -> (-100.7493, -63.5)
  line L596 (-106.2485, -73.025) -> (-100.7493, -82.55)
  line L597 (-100.7493, -63.5) -> (-106.2485, -73.025)
  line L598 (-119.9967, -93.6625) -> (-108.9982, -93.6625)
  line L599 (-108.9982, -93.6625) -> (-103.4989, -84.1375)
  line L600 (-103.4989, -84.1375) -> (-108.9982, -74.6125)
  line L601 (-108.9982, -74.6125) -> (-119.9967, -74.6125)
  line L602 (-125.4959, -84.1375) -> (-119.9967, -93.6625)
  line L603 (-119.9967, -74.6125) -> (-125.4959, -84.1375)
  line L604 (-139.2441, -104.775) -> (-128.2456, -104.775)
  line L605 (-128.2456, -104.775) -> (-122.7463, -95.25)
  line L606 (-122.7463, -95.25) -> (-128.2456, -85.725)
  line L607 (-128.2456, -85.725) -> (-139.2441, -85.725)
  line L608 (-144.7434, -95.25) -> (-139.2441, -104.775)
  line L609 (-139.2441, -85.725) -> (-144.7434, -95.25)
  line L610 (-158.4915, -115.8875) -> (-147.493, -115.8875)
  line L611 (-147.493, -115.8875) -> (-141.9937, -106.3625)
  line L612 (-141.9937, -106.3625) -> (-147.493, -96.8375)
  line L613 (-147.493, -96.8375) -> (-158.4915, -96.8375)
  line L614 (-163.9908, -106.3625) -> (-158.4915, -115.8875)
  line L615 (-158.4915, -96.8375) -> (-163.9908, -106.3625)
  line L616 (-177.7389, -127) -> (-166.7404, -127)
  line L617 (-166.7404, -127) -> (-161.2411, -117.475)
  line L618 (-161.2411, -117.475) -> (-166.7404, -107.95)
  line L619 (-166.7404, -107.95) -> (-177.7389, -107.95)
  line L620 (-183.2382, -117.475) -> (-177.7389, -127)
  line L621 (-177.7389, -107.95) -> (-183.2382, -117.475)
  line L622 (-196.9863, -138.1125) -> (-185.9878, -138.1125)
  line L623 (-185.9878, -138.1125) -> (-180.4886, -128.5875)
  line L624 (-180.4886, -128.5875) -> (-185.9878, -119.0625)
  line L625 (-185.9878, -119.0625) -> (-196.9863, -119.0625)
  line L626 (-202.4856, -128.5875) -> (-196.9863, -138.1125)
  line L627 (-196.9863, -119.0625) -> (-202.4856, -128.5875)
  line L628 (-216.2337, -149.225) -> (-205.2352, -149.225)
  line L629 (-205.2352, -149.225) -> (-199.736, -139.7)
  line L630 (-199.736, -139.7) -> (-205.2352, -130.175)
  line L631 (-205.2352, -130.175) -> (-216.2337, -130.175)
  line L632 (-221.733, -139.7) -> (-216.2337, -149.225)
  line L633 (-216.2337, -130.175) -> (-221.733, -139.7)
  line L634 (-235.4812, -160.3375) -> (-224.4826, -160.3375)
  line L635 (-224.4826, -160.3375) -> (-218.9834, -150.8125)
  line L636 (-218.9834, -150.8125) -> (-224.4826, -141.2875)
  line L637 (-224.4826, -141.2875) -> (-235.4812, -141.2875)
  line L638 (-240.9804, -150.8125) -> (-235.4812, -160.3375)
  line L639 (-235.4812, -141.2875) -> (-240.9804, -150.8125)
  line L640 (-254.7286, -171.45) -> (-243.7301, -171.45)
  line L641 (-243.7301, -171.45) -> (-238.2308, -161.925)
  line L642 (-238.2308, -161.925) -> (-243.7301, -152.4)
  line L643 (-243.7301, -152.4) -> (-254.7286, -152.4)
  line L644 (-260.2278, -161.925) -> (-254.7286, -171.45)
  line L645 (-254.7286, -152.4) -> (-260.2278, -161.925)
  line L646 (33.9826, -26.9875) -> (44.9812, -26.9875)
  line L647 (44.9812, -26.9875) -> (50.4804, -17.4625)
  line L648 (50.4804, -17.4625) -> (44.9812, -7.9375)
  line L649 (44.9812, -7.9375) -> (33.9826, -7.9375)
  line L650 (28.4834, -17.4625) -> (33.9826, -26.9875)
  line L651 (33.9826, -7.9375) -> (28.4834, -17.4625)
  line L652 (14.7352, -38.1) -> (25.7337, -38.1)
  line L653 (25.7337, -38.1) -> (31.233, -28.575)
  line L654 (31.233, -28.575) -> (25.7337, -19.05)
  line L655 (25.7337, -19.05) -> (14.7352, -19.05)
  line L656 (9.236, -28.575) -> (14.7352, -38.1)
  line L657 (14.7352, -19.05) -> (9.236, -28.575)
  line L658 (-4.5122, -49.2125) -> (6.4863, -49.2125)
  line L659 (6.4863, -49.2125) -> (11.9856, -39.6875)
  line L660 (11.9856, -39.6875) -> (6.4863, -30.1625)
  line L661 (6.4863, -30.1625) -> (-4.5122, -30.1625)
  line L662 (-10.0114, -39.6875) -> (-4.5122, -49.2125)
  line L663 (-4.5122, -30.1625) -> (-10.0114, -39.6875)
  line L664 (-23.7596, -60.325) -> (-12.7611, -60.325)
  line L665 (-12.7611, -60.325) -> (-7.2618, -50.8)
  line L666 (-7.2618, -50.8) -> (-12.7611, -41.275)
  line L667 (-12.7611, -41.275) -> (-23.7596, -41.275)
  line L668 (-29.2589, -50.8) -> (-23.7596, -60.325)
  line L669 (-23.7596, -41.275) -> (-29.2589, -50.8)
  line L670 (-43.007, -71.4375) -> (-32.0085, -71.4375)
  line L671 (-32.0085, -71.4375) -> (-26.5092, -61.9125)
  line L672 (-26.5092, -61.9125) -> (-32.0085, -52.3875)
  line L673 (-32.0085, -52.3875) -> (-43.007, -52.3875)
  line L674 (-48.5063, -61.9125) -> (-43.007, -71.4375)
  line L675 (-43.007, -52.3875) -> (-48.5063, -61.9125)
  line L676 (-62.2544, -82.55) -> (-51.2559, -82.55)
  line L677 (-51.2559, -82.55) -> (-45.7566, -73.025)
  line L678 (-45.7566, -73.025) -> (-51.2559, -63.5)
  line L679 (-51.2559, -63.5) -> (-62.2544, -63.5)
  line L680 (-67.7537, -73.025) -> (-62.2544, -82.55)
  line L681 (-62.2544, -63.5) -> (-67.7537, -73.025)
  line L682 (-81.5018, -93.6625) -> (-70.5033, -93.6625)
  line L683 (-70.5033, -93.6625) -> (-65.0041, -84.1375)
  line L684 (-65.0041, -84.1375) -> (-70.5033, -74.6125)
  line L685 (-70.5033, -74.6125) -> (-81.5018, -74.6125)
  line L686 (-87.0011, -84.1375) -> (-81.5018, -93.6625)
  line L687 (-81.5018, -74.6125) -> (-87.0011, -84.1375)
  line L688 (-119.9967, -115.8875) -> (-108.9982, -115.8875)
  line L689 (-108.9982, -115.8875) -> (-103.4989, -106.3625)
  line L690 (-103.4989, -106.3625) -> (-108.9982, -96.8375)
  line L691 (-108.9982, -96.8375) -> (-119.9967, -96.8375)
  line L692 (-125.4959, -106.3625) -> (-119.9967, -115.8875)
  line L693 (-119.9967, -96.8375) -> (-125.4959, -106.3625)
  line L694 (-139.2441, -127) -> (-128.2456, -127)
  line L695 (-128.2456, -127) -> (-122.7463, -117.475)
  line L696 (-122.7463, -117.475) -> (-128.2456, -107.95)
  line L697 (-128.2456, -107.95) -> (-139.2441, -107.95)
  line L698 (-144.7434, -117.475) -> (-139.2441, -127)
  line L699 (-139.2441, -107.95) -> (-144.7434, -117.475)
  line L700 (-158.4915, -138.1125) -> (-147.493, -138.1125)
  line L701 (-147.493, -138.1125) -> (-141.9937, -128.5875)
  line L702 (-141.9937, -128.5875) -> (-147.493, -119.0625)
  line L703 (-147.493, -119.0625) -> (-158.4915, -119.0625)
  line L704 (-163.9908, -128.5875) -> (-158.4915, -138.1125)
  line L705 (-158.4915, -119.0625) -> (-163.9908, -128.5875)
  line L706 (-177.7389, -149.225) -> (-166.7404, -149.225)
  line L707 (-166.7404, -149.225) -> (-161.2411, -139.7)
  line L708 (-161.2411, -139.7) -> (-166.7404, -130.175)
  line L709 (-166.7404, -130.175) -> (-177.7389, -130.175)
  line L710 (-183.2382, -139.7) -> (-177.7389, -149.225)
  line L711 (-177.7389, -130.175) -> (-183.2382, -139.7)
  line L712 (-196.9863, -160.3375) -> (-185.9878, -160.3375)
  line L713 (-185.9878, -160.3375) -> (-180.4886, -150.8125)
  line L714 (-180.4886, -150.8125) -> (-185.9878, -141.2875)
  line L715 (-185.9878, -141.2875) -> (-196.9863, -141.2875)
  line L716 (-202.4856, -150.8125) -> (-196.9863, -160.3375)
  line L717 (-196.9863, -141.2875) -> (-202.4856, -150.8125)
  line L718 (-216.2337, -171.45) -> (-205.2352, -171.45)
  line L719 (-205.2352, -171.45) -> (-199.736, -161.925)
  line L720 (-199.736, -161.925) -> (-205.2352, -152.4)
  line L721 (-205.2352, -152.4) -> (-216.2337, -152.4)
  line L722 (-221.733, -161.925) -> (-216.2337, -171.45)
  line L723 (-216.2337, -152.4) -> (-221.733, -161.925)
  line L724 (-235.4812, -182.5625) -> (-224.4826, -182.5625)
  line L725 (-224.4826, -182.5625) -> (-218.9834, -173.0375)
  line L726 (-218.9834, -173.0375) -> (-224.4826, -163.5125)
  line L727 (-224.4826, -163.5125) -> (-235.4812, -163.5125)
  line L728 (-240.9804, -173.0375) -> (-235.4812, -182.5625)
  line L729 (-235.4812, -163.5125) -> (-240.9804, -173.0375)
  line L730 (53.2301, -38.1) -> (64.2286, -38.1)
  line L731 (64.2286, -38.1) -> (69.7278, -28.575)
  line L732 (69.7278, -28.575) -> (64.2286, -19.05)
  line L733 (64.2286, -19.05) -> (53.2301, -19.05)
  line L734 (47.7308, -28.575) -> (53.2301, -38.1)
  line L735 (53.2301, -19.05) -> (47.7308, -28.575)
  line L736 (33.9826, -49.2125) -> (44.9812, -49.2125)
  line L737 (44.9812, -49.2125) -> (50.4804, -39.6875)
  line L738 (50.4804, -39.6875) -> (44.9812, -30.1625)
  line L739 (44.9812, -30.1625) -> (33.9826, -30.1625)
  line L740 (28.4834, -39.6875) -> (33.9826, -49.2125)
  line L741 (33.9826, -30.1625) -> (28.4834, -39.6875)
  line L742 (14.7352, -60.325) -> (25.7337, -60.325)
  line L743 (25.7337, -60.325) -> (31.233, -50.8)
  line L744 (31.233, -50.8) -> (25.7337, -41.275)
  line L745 (25.7337, -41.275) -> (14.7352, -41.275)
  line L746 (9.236, -50.8) -> (14.7352, -60.325)
  line L747 (14.7352, -41.275) -> (9.236, -50.8)
  line L748 (-4.5122, -71.4375) -> (6.4863, -71.4375)
  line L749 (6.4863, -71.4375) -> (11.9856, -61.9125)
  line L750 (11.9856, -61.9125) -> (6.4863, -52.3875)
  line L751 (6.4863, -52.3875) -> (-4.5122, -52.3875)
  line L752 (-10.0114, -61.9125) -> (-4.5122, -71.4375)
  line L753 (-4.5122, -52.3875) -> (-10.0114, -61.9125)
  line L754 (-23.7596, -82.55) -> (-12.7611, -82.55)
  line L755 (-12.7611, -82.55) -> (-7.2618, -73.025)
  line L756 (-7.2618, -73.025) -> (-12.7611, -63.5)
  line L757 (-12.7611, -63.5) -> (-23.7596, -63.5)
  line L758 (-29.2589, -73.025) -> (-23.7596, -82.55)
  line L759 (-23.7596, -63.5) -> (-29.2589, -73.025)
  line L760 (-43.007, -93.6625) -> (-32.0085, -93.6625)
  line L761 (-32.0085, -93.6625) -> (-26.5092, -84.1375)
  line L762 (-26.5092, -84.1375) -> (-32.0085, -74.6125)
  line L763 (-32.0085, -74.6125) -> (-43.007, -74.6125)
  line L764 (-48.5063, -84.1375) -> (-43.007, -93.6625)
  line L765 (-43.007, -74.6125) -> (-48.5063, -84.1375)
  line L766 (-62.2544, -104.775) -> (-51.2559, -104.775)
  line L767 (-51.2559, -104.775) -> (-45.7566, -95.25)
  line L768 (-45.7566, -95.25) -> (-51.2559, -85.725)
  line L769 (-51.2559, -85.725) -> (-62.2544, -85.725)
  line L770 (-67.7537, -95.25) -> (-62.2544, -104.775)
  line L771 (-62.2544, -85.725) -> (-67.7537, -95.25)
  line L772 (-81.5018, -115.8875) -> (-70.5033, -115.8875)
  line L773 (-70.5033, -115.8875) -> (-65.0041, -106.3625)
  line L774 (-65.0041, -106.3625) -> (-70.5033, -96.8375)
  line L775 (-70.5033, -96.8375) -> (-81.5018, -96.8375)
  line L776 (-87.0011, -106.3625) -> (-81.5018, -115.8875)
  line L777 (-81.5018, -96.8375) -> (-87.0011, -106.3625)
  line L778 (-100.7493, -127) -> (-89.7507, -127)
  line L779 (-89.7507, -127) -> (-84.2515, -117.475)
  line L780 (-84.2515, -117.475) -> (-89.7507, -107.95)
  line L781 (-89.7507, -107.95) -> (-100.7493, -107.95)
  line L782 (-106.2485, -117.475) -> (-100.7493, -127)
  line L783 (-100.7493, -107.95) -> (-106.2485, -117.475)
  line L784 (-119.9967, -138.1125) -> (-108.9982, -138.1125)
  line L785 (-108.9982, -138.1125) -> (-103.4989, -128.5875)
  line L786 (-103.4989, -128.5875) -> (-108.9982, -119.0625)
  line L787 (-108.9982, -119.0625) -> (-119.9967, -119.0625)
  line L788 (-125.4959, -128.5875) -> (-119.9967, -138.1125)
  line L789 (-119.9967, -119.0625) -> (-125.4959, -128.5875)
  line L790 (-139.2441, -149.225) -> (-128.2456, -149.225)
  line L791 (-128.2456, -149.225) -> (-122.7463, -139.7)
  line L792 (-122.7463, -139.7) -> (-128.2456, -130.175)
  line L793 (-128.2456, -130.175) -> (-139.2441, -130.175)
  line L794 (-144.7434, -139.7) -> (-139.2441, -149.225)
  line L795 (-139.2441, -130.175) -> (-144.7434, -139.7)
  line L796 (-158.4915, -160.3375) -> (-147.493, -160.3375)
  line L797 (-147.493, -160.3375) -> (-141.9937, -150.8125)
  line L798 (-141.9937, -150.8125) -> (-147.493, -141.2875)
  line L799 (-147.493, -141.2875) -> (-158.4915, -141.2875)
  line L800 (-163.9908, -150.8125) -> (-158.4915, -160.3375)
  line L801 (-158.4915, -141.2875) -> (-163.9908, -150.8125)
  line L802 (-177.7389, -171.45) -> (-166.7404, -171.45)
  line L803 (-166.7404, -171.45) -> (-161.2411, -161.925)
  line L804 (-161.2411, -161.925) -> (-166.7404, -152.4)
  line L805 (-166.7404, -152.4) -> (-177.7389, -152.4)
  line L806 (-183.2382, -161.925) -> (-177.7389, -171.45)
  line L807 (-177.7389, -152.4) -> (-183.2382, -161.925)
  line L808 (-196.9863, -182.5625) -> (-185.9878, -182.5625)
  line L809 (-185.9878, -182.5625) -> (-180.4886, -173.0375)
  line L810 (-180.4886, -173.0375) -> (-185.9878, -163.5125)
  line L811 (-185.9878, -163.5125) -> (-196.9863, -163.5125)
  line L812 (-202.4856, -173.0375) -> (-196.9863, -182.5625)
  line L813 (-196.9863, -163.5125) -> (-202.4856, -173.0375)
  line L814 (-216.2337, -193.675) -> (-205.2352, -193.675)
  line L815 (-205.2352, -193.675) -> (-199.736, -184.15)
  line L816 (-199.736, -184.15) -> (-205.2352, -174.625)
  line L817 (-205.2352, -174.625) -> (-216.2337, -174.625)
  line L818 (-221.733, -184.15) -> (-216.2337, -193.675)
  line L819 (-216.2337, -174.625) -> (-221.733, -184.15)
  line L820 (72.4775, -49.2125) -> (83.476, -49.2125)
  line L821 (83.476, -49.2125) -> (88.9753, -39.6875)
  line L822 (88.9753, -39.6875) -> (83.476, -30.1625)
  line L823 (83.476, -30.1625) -> (72.4775, -30.1625)
  line L824 (66.9782, -39.6875) -> (72.4775, -49.2125)
  line L825 (72.4775, -30.1625) -> (66.9782, -39.6875)
  line L826 (53.2301, -60.325) -> (64.2286, -60.325)
  line L827 (64.2286, -60.325) -> (69.7278, -50.8)
  line L828 (69.7278, -50.8) -> (64.2286, -41.275)
  line L829 (64.2286, -41.275) -> (53.2301, -41.275)
  line L830 (47.7308, -50.8) -> (53.2301, -60.325)
  line L831 (53.2301, -41.275) -> (47.7308, -50.8)
  line L832 (33.9826, -71.4375) -> (44.9812, -71.4375)
  line L833 (44.9812, -71.4375) -> (50.4804, -61.9125)
  line L834 (50.4804, -61.9125) -> (44.9812, -52.3875)
  line L835 (44.9812, -52.3875) -> (33.9826, -52.3875)
  line L836 (28.4834, -61.9125) -> (33.9826, -71.4375)
  line L837 (33.9826, -52.3875) -> (28.4834, -61.9125)
  line L838 (14.7352, -82.55) -> (25.7337, -82.55)
  line L839 (25.7337, -82.55) -> (31.233, -73.025)
  line L840 (31.233, -73.025) -> (25.7337, -63.5)
  line L841 (25.7337, -63.5) -> (14.7352, -63.5)
  line L842 (9.236, -73.025) -> (14.7352, -82.55)
  line L843 (14.7352, -63.5) -> (9.236, -73.025)
  line L844 (-4.5122, -93.6625) -> (6.4863, -93.6625)
  line L845 (6.4863, -93.6625) -> (11.9856, -84.1375)
  line L846 (11.9856, -84.1375) -> (6.4863, -74.6125)
  line L847 (6.4863, -74.6125) -> (-4.5122, -74.6125)
  line L848 (-10.0114, -84.1375) -> (-4.5122, -93.6625)
  line L849 (-4.5122, -74.6125) -> (-10.0114, -84.1375)
  line L850 (-23.7596, -104.775) -> (-12.7611, -104.775)
  line L851 (-12.7611, -104.775) -> (-7.2618, -95.25)
  line L852 (-7.2618, -95.25) -> (-12.7611, -85.725)
  line L853 (-12.7611, -85.725) -> (-23.7596, -85.725)
  line L854 (-29.2589, -95.25) -> (-23.7596, -104.775)
  line L855 (-23.7596, -85.725) -> (-29.2589, -95.25)
  line L856 (-43.007, -115.8875) -> (-32.0085, -115.8875)
  line L857 (-32.0085, -115.8875) -> (-26.5092, -106.3625)
  line L858 (-26.5092, -106.3625) -> (-32.0085, -96.8375)
  line L859 (-32.0085, -96.8375) -> (-43.007, -96.8375)
  line L860 (-48.5063, -106.3625) -> (-43.007, -115.8875)
  line L861 (-43.007, -96.8375) -> (-48.5063, -106.3625)
  line L862 (-62.2544, -127) -> (-51.2559, -127)
  line L863 (-51.2559, -127) -> (-45.7566, -117.475)
  line L864 (-45.7566, -117.475) -> (-51.2559, -107.95)
  line L865 (-51.2559, -107.95) -> (-62.2544, -107.95)
  line L866 (-67.7537, -117.475) -> (-62.2544, -127)
  line L867 (-62.2544, -107.95) -> (-67.7537, -117.475)
  line L868 (-81.5018, -138.1125) -> (-70.5033, -138.1125)
  line L869 (-70.5033, -138.1125) -> (-65.0041, -128.5875)
  line L870 (-65.0041, -128.5875) -> (-70.5033, -119.0625)
  line L871 (-70.5033, -119.0625) -> (-81.5018, -119.0625)